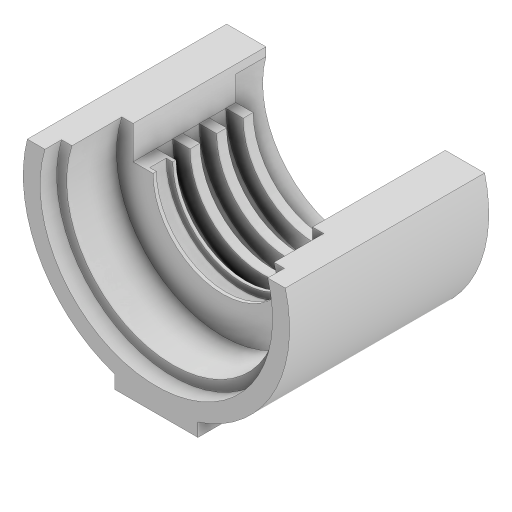
# Autodesk Inventor part: HAL-filter-holder1
Saved by Autodesk Inventor 2023 (Build 270158000, 158)
## iProperties
Created: 2023-10-11
Part Number: HAL-filter-holder1
Material: Generic
Document SubType Name: Modeling
Designer: spim-user
Density: 1 g/cm^3
Appearance: Default
Author: spim-user
Autodesk Inventor part; units mm, degrees
ref_plane "YZ Plane" through (0, 0, 0) normal (1, 0, 0) x (0, 1, 0)
ref_plane "XZ Plane" through (0, 0, 0) normal (0, 1, 0) x (-1, 0, 0)
ref_plane "XY Plane" through (0, 0, 0) normal (0, 0, 1) x (1, 0, 0)
sketch "Sketch1" plane through (0, 0, 0) normal (0, 1, 0) x (-1, 0, 0)
  line L0 (-35, 10) -> (-40.1, 10)
  line L1 (-40.1, 10) -> (-40.1, -50)
  line L2 (-40.1, -50) -> (-35.1, -50)
  line L3 (-35, 5) -> (-32, 5)
  line L4 (-32, 5) -> (-32, -10)
  line L5 (-32, -10) -> (-23, -10)
  line L6 (-23, -11) -> (-23, -15.9282)
  line L7 (-22, -16.9282) -> (-27, -16.9282)
  line L8 (-27, -16.9282) -> (-27, -21.9282)
  line L9 (-27, -21.9282) -> (-21.8, -21.9282)
  line L10 (-21.8, -21.9282) -> (-21.8, -24.9282)
  line L11 (-21.8, -24.9282) -> (-27, -24.9282)
  line L12 (-27, -24.9282) -> (-27, -29.9282)
  line L13 (-27, -29.9282) -> (-21.8, -29.9282)
  line L14 (-21.8, -29.9282) -> (-21.8, -32.9282)
  line L15 (-21.8, -32.9282) -> (-27, -32.9282)
  line L16 (-27, -32.9282) -> (-27, -37.9282)
  line L17 (-27, -37.9282) -> (-21.8, -37.9282)
  line L18 (-21.8, -37.9282) -> (-21.8, -40.9282)
  line L19 (-21.8, -40.9282) -> (-28, -40.9282)
  line L20 (-23, -10) -> (-21, -10)
  line L21 (-21, -10) -> (-21, -11)
  line L22 (-21, -11) -> (-23, -11)
  line L23 (-22, -16.9282) -> (-21, -16.9282)
  line L24 (-21, -16.9282) -> (-21, -15.9282)
  line L25 (-21, -15.9282) -> (-23, -15.9282)
  line L26 (-28, -40.9282) -> (-28, -50)
  line L27 (-28, -50) -> (-35.1, -50)
  line L28 (-35, 5) -> (-35, 10)
  line L29 (0, -62) -> (0, 22) projected
  point P0 (0, 0)
  point P1 (-33.5, 5)
  dimension "d4" = 3
  dimension "d6" = 23
  dimension "d7" = 5
  dimension "d8" = 5
  dimension "d11" = 3
  dimension "d12" = 5
  dimension "d13" = 3
  dimension "d14" = 5
  dimension "d15" = 3
  dimension "d16" = 2
  dimension "d17" = 1
  dimension "d18" = 1
  dimension "d19" = 28
  dimension "d20" = 27
  dimension "d21" = 27
  dimension "d22" = 23
  dimension "d28" = 15
  dimension "d29" = 5
  dimension "d30" = 32
  constraints: 58 end point, 18 perpendicular, 8 point on line, 4 parallel, 3 horizontal, 2 vertical, 1 midpoint
  measures "d4" distance of L3.start L3.end
  measures "d6" horizontal distance of L5.end point (0, 0)
  measures "d7" distance of L7.start L7.end
  measures "d8" distance of L7.end L8.end
  measures "d11" distance of L9.end L10.end
  measures "d12" distance of L11.end L12.end
  measures "d13" distance of L13.end L14.end
  measures "d14" distance of L15.end L16.end
  measures "d15" distance of L17.end L18.end
  measures "d16" distance of L5.end L20.end
  measures "d17" distance of L20.end L21.end
  measures "d18" distance of L23.end L24.end
  measures "d19" distance from line of L26 point (0, 0)
  measures "d20" distance from line of L16 point (0, 0)
  measures "d21" distance from line of L8 point (0, 0)
  measures "d22" distance from line of L6 point (0, 0)
  measures "d28" distance from line of point (-33.5, 5) L5
  measures "d29" distance between parallel lines of L0 L3
  measures "d30" distance between parallel lines of L4 L29
revolve "Revolution1" add sketch "Sketch1" angle 360 about axis through (0, 0, -10) along (0, 0, 1)
sketch "Sketch2" plane through (0, 0, 10) normal (0, 0, 1) x (1, 0, 0)
  line L0 (-41.9384, 10) -> (42.6332, 10)
  line L1 (42.6332, 10) -> (42.6332, 41.1939)
  line L2 (42.6332, 41.1939) -> (-41.9384, 41.1939)
  line L3 (-41.9384, 41.1939) -> (-41.9384, 10)
  point P0 (0, 0)
  constraints: 8 end point, 2 parallel, 1 horizontal, 1 perpendicular
extrude "Extrusion1" cut sketch "Sketch2" against normal through all
sketch "Sketch3" plane through (0, 0, -10) normal (0, 0, 1) x (1, 0, 0)
  arc A0 (-25.0799, 10) -> (25.0799, 10) centre (0, 0) ccw projected
  line L0 (-27, 0) -> (27, 0)
  line L1 (27, 0) -> (27, 40.4991)
  line L2 (27, 40.4991) -> (-27, 40.4991)
  line L3 (-27, 40.4991) -> (-27, 0)
  constraints: 8 end point, 2 parallel, 1 horizontal, 1 perpendicular, 1 point on circle
extrude "Extrusion2" cut sketch "Sketch3" against normal through all contours L3 L2 L1 L0
sketch "Sketch4" plane through (0, 0, 10) normal (0, 0, 1) x (1, 0, 0)
  arc A0 (-38.8331, 10) -> (38.8331, 10) centre (0, 0) ccw projected
  line L0 (12.5184, -42.1041) -> (-12.5184, -42.1041)
  line L1 (-12.5184, -42.1041) -> (-12.5184, -38.0959)
  line L2 (-12.5184, -38.0959) -> (12.5184, -38.0959)
  line L3 (12.5184, -38.0959) -> (12.5184, -42.1041)
  line L4 (12.5184, -42.1041) -> (-12.5184, -38.0959) construction
  line L5 (-12.5184, -42.1041) -> (12.5184, -38.0959) construction
  point P0 (0, -40.1)
  constraints: 12 end point, 2 midpoint, 2 parallel, 2 point on circle, 1 horizontal, 1 perpendicular
extrude "Extrusion3" add sketch "Sketch4" against normal up to surface (60 mm away)
body "Solid1"
